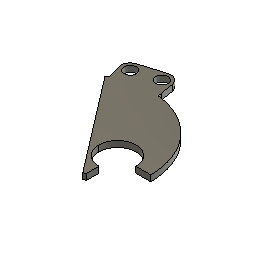
microwave motor spacer and adapter v1 (Autodesk Fusion 360 design; units mm, degrees)
Autodesk Fusion 360 part; units mm, degrees
sketch "Sketch1" plane through (0, 0, 0) normal (0, 1, 0) x (1, 0, 0)
  circle A0 centre (0, 0) radius 24
  line L0 (0, 0) -> (6.875, 0)
  circle A1 centre (13, 0.0099) radius 6.125
  line L1 (6.875, 0) -> (6.875, 22.9942)
  line L2 (6.875, 0) -> (2.6694, 23.8511)
  line L3 (6.875, 0) -> (31.2042, 0) construction
  line L4 (6.875, 0) -> (-11.0165, 21.3222)
  line L5 (2.6694, 23.8511) -> (2.4763, 24.9554)
  line L6 (2.4763, 24.9554) -> (1.6749, 29.5003)
  line L7 (-11.0165, 21.3222) -> (-12.2065, 25.7634)
  line L8 (-11.0165, 21.3222) -> (-3.4291, 21.3222) construction
  line L9 (-10.1808, 29.4103) -> (-2.1517, 31.8498)
  arc A2 (-10.1808, 29.4103) -> (-12.2065, 25.7634) centre (-9.3087, 26.5399) ccw
  arc A3 (1.6749, 29.5003) -> (-2.1517, 31.8498) centre (-1.2795, 28.9794) ccw
  line L10 (-15.8784, 27.6774) -> (17.6976, -16.2109)
  circle A4 centre (-9.3087, 26.5399) radius 2
  circle A5 centre (-1.2795, 28.9794) radius 2
  line L11 (13, 0.0099) -> (19.125, 0)
  line L12 (13, 0.0099) -> (13, -6.1151)
  line L13 (13, -6.1151) -> (13, -10.0705)
  line L14 (19.125, 0) -> (24, 0)
  point P0 (1.0871, 32.8338)
  point P1 (-12.9576, 28.5667)
  dimension "d1" = 48
  dimension "d2" = 6.875
  dimension "d4" = 12.25
  dimension "d5" = 100
  dimension "d6" = 130
  dimension "d7" = 8
  dimension "d8" = 105
  dimension "d9" = 7.5
  dimension "d10" = 3
  dimension "d11" = 3
  dimension "d12" = 4
  dimension "d13" = 4
  constraint coincident A0.centre L0.start
  constraint horizontal L0
  constraint coincident A0 L1.end
  constraint tangent A1 L1
  constraint perpendicular L0 L1
  constraint horizontal L3
  constraint coincident A0 L2.end
  constraint coincident A0 L4.end
  constraint parallel L2 L6
  constraint horizontal L8
  constraint coincident P1 L7
  constraint coincident P1 L9
  constraint tangent L7 A2
  constraint tangent L9 A2
  constraint coincident P0 L9
  constraint coincident P0 L6
  constraint tangent L9 A3
  constraint tangent L6 A3
  constraint tangent A1 L10
  constraint coincident L4.end L10
  constraint coincident A0 L10.end
  constraint concentric A2 A4
  constraint concentric A3 A5
  constraint coincident A1.centre L11.start
  constraint coincident L3 L11.end
  constraint coincident A1 L11.end
  constraint coincident A1 L12.end
  constraint perpendicular L3 L12
  constraint coincident L10 L13.end
  constraint parallel L12 L13
  constraint coincident A0 L14.end
  constraint coincident L3 L14.end
  measures "d1" diameter of A0
  measures "d2" distance of A0.centre L0.end
  measures "d4" diameter of A1
  measures "d5" angle of L2 L3
  measures "d6" angle of L3 L4
  measures "d7" distance of L5.end P0
  measures "d8" angle of L7 L8
  measures "d9" distance of L4.end P1
  measures "d10" radius of A2
  measures "d11" radius of A3
  measures "d12" diameter of A4
  measures "d13" diameter of A5
extrude "Extrude1" add sketch "Sketch1" along normal blind 2 contours L0 A1 L10 | L0 L4 L10 | A0 L2 L4 | A0 A1 L1 L14 | A0 L1 L2 | A0 L5 L6 L7 L9 A2 A3 | A1 L10 L13
extrude "Extrude2" add 2 faces at (9.7569, 1.3333, 5.8313) (-4.6325, 0.6667, -12.9776) along direction (-0.794233, 0, 0.607614) blind 1
